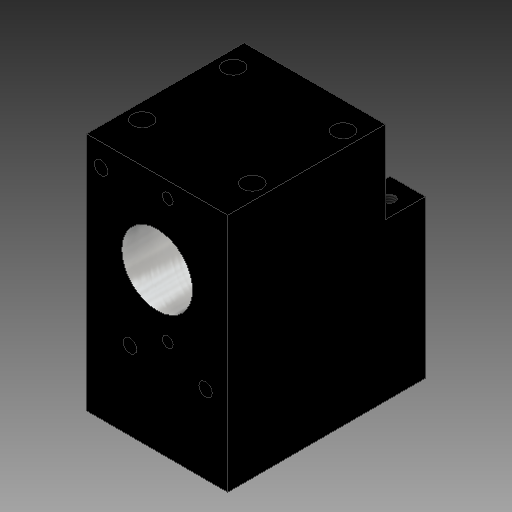
# Autodesk Inventor part: J007515
Saved by Autodesk Inventor 2018.2 (Build 222227000, 227)
## iProperties
Created: 2018-06-06
Part Number: J007515
Material: ALUMINUM, 6061-T651
Document SubType Name: Modeling
Designer: legant_local
Density: 2.7 g/cm^3
Appearance: Anodized - Black
Catalog Web Link: MPFI custom
Description: ResGalvoMount_wobble
Vendor: HHMI: JRC - JET
Project: P-303502
ALTERED ITEM PART NUMBER: N/A
ALTERED ITEM VENDOR: N/A
ALTERED ITEM DESCRIPTION: N/A
DESIGN DEPARTMENT: HHMI: JRC - ID&F
LAB/DEPT: BETZIG (LAB)
REQUESTING SCIENTIST: BETZIG, ERIC
SPECIAL FINISH: ANODIZE PER MIL-A-8625F, TYPE II, CLASS 2 (BLACK)
SURFACE ROUGHNESS: 32 Ra
Author: legant_local
Revision Number: 0
Autodesk Inventor part; units mm, degrees
ref_plane "YZ Plane" through (0, 0, 0) normal (1, 0, 0) x (0, 1, 0)
ref_plane "XZ Plane" through (0, 0, 0) normal (0, 1, 0) x (-1, 0, 0)
ref_plane "XY Plane" through (0, 0, 0) normal (0, 0, 1) x (1, 0, 0)
sketch "Sketch1" plane through (0, 0, 0) normal (0, 0, 1) x (1, 0, 0)
  line L0 (-15.875, 18.975) -> (15.875, 18.975)
  line L1 (15.875, 18.975) -> (15.875, -35)
  line L2 (15.875, -35) -> (-15.875, -35)
  line L3 (-15.875, -35) -> (-15.875, 18.975)
  point P0 (0, 0)
  dimension "d0" = 31.75
  dimension "d1" = 53.975
  dimension "d3" = 35
  dimension "d4" = 15.875
  constraints: 8 end point, 2 parallel, 1 horizontal, 1 perpendicular
  measures "d0" distance of L1.end L2.end
  measures "d1" distance of L0.end L1.end
  measures "d3" distance from line of L2 point (0, 0)
  measures "d4" distance from line of L3 point (0, 0)
extrude "Extrusion1" add sketch "Sketch1" along normal blind 44.45
sketch "Sketch2" plane through (0, 0, 44.45) normal (0, 0, 1) x (1, 0, 0)
  circle A0 centre (0, 0.3862) radius 7.9629
  line L0 (15.875, 18.975) -> (-15.875, 18.975) projected
  line L1 (-15.875, 18.975) -> (-15.875, -35) projected
  line L2 (-15.875, -35) -> (15.875, -35) projected
  line L3 (15.875, -35) -> (15.875, 18.975) projected
  line L4 (15.875, 18.975) -> (-15.875, 18.975) projected
  line L5 (0, 18.975) -> (0, -35) construction
  dimension "d7" = 15.9258
  dimension "d124" = 35.3862
  constraints: 2 end point, 2 midpoint, 1 centre point, 1 point on line
  measures "d7" diameter of A0
  measures "d124" distance from line of L2 A0.centre
extrude "Extrusion2" cut sketch "Sketch2" against normal through all contours A0
sketch "Sketch4" plane through (-15.875, 18.975, 0) normal (0, 1, 0) x (1, 0, 0)
  line L0 (0, 0) -> (31.75, 0) projected
  line L1 (31.75, 0) -> (0, 0)
  line L2 (0, 0) -> (0, -9)
  line L3 (0, -9) -> (31.75, -9)
  line L4 (31.75, -9) -> (31.75, 0)
  line L5 (0, 0) -> (0, -44.45) projected
  point P0 (15.875, 0)
  point P1 (0, -4.5)
  dimension "d15" = 9
  constraints: 8 end point, 2 parallel, 1 horizontal, 1 midpoint, 1 perpendicular, 1 point on line
  measures "d15" distance of L3.end L0.end
extrude "Extrusion4" cut sketch "Sketch4" against normal blind 18.5888
sketch "Sketch6" plane through (0, 0, 44.45) normal (0, 0, 1) x (1, 0, 0)
  line L0 (15.875, -15.95) -> (-11.125, -15.95) projected
  line L1 (-11.125, -15.95) -> (-11.125, 18.975) projected
  point P0 (0, 0)
  point P1 (-6.125, -17.45)
  point P2 (10.875, -17.45)
  point P3 (-12.625, 13.975)
  dimension "d33" = 1.5
  dimension "d34" = 1.5
  dimension "d35" = 5
  dimension "d36" = 5
  dimension "d44" = 5
  dimension "d45" = 1.5
  measures "d33" distance from line of L0 point (10.875, -17.45)
  measures "d34" distance from line of L0 point (-6.125, -17.45)
  measures "d35" horizontal distance of point (-6.125, -17.45) L0.end
  measures "d36" horizontal distance of L0.start point (10.875, -17.45)
  measures "d44" vertical distance of L1.end point (-12.625, 13.975)
  measures "d45" distance from line of L1 point (-12.625, 13.975)
hole "Press fit for D3mm_L10mm Dowel - pin to protrude 5mm" at (-6.125, -17.45, 44.45) at (10.875, -17.45, 44.45) at (-12.625, 13.975, 44.45) direction (0, 0, -1) diameter 3 depth 5 tip angle 118
sketch "Sketch9" plane through (-15.875, 18.975, 44.45) normal (0, 1, 0) x (1, 0, 0)
  line L0 (31.75, 35.45) -> (0, 35.45) projected
  line L1 (0, 35.45) -> (0, 0) projected
  line L2 (31.75, 0) -> (0, 0) projected
  line L3 (31.75, 35.45) -> (31.75, 0) projected
  line L4 (23.8379, 35.45) -> (23.8379, 44.45) projected
  line L5 (7.9121, 44.45) -> (23.8379, 44.45) projected
  line L6 (7.9121, 44.45) -> (7.9121, 35.45) projected
  line L7 (7.9121, 35.45) -> (23.8379, 35.45) projected
  line L8 (23.8379, 0) -> (7.9121, 0) projected
  point P0 (15.875, 44.45)
  point P1 (28.25, 9)
  point P2 (3.5, 9)
  point P3 (3.5, 29.45)
  point P4 (28.25, 29.45)
  dimension "d60" = 9
  dimension "d61" = 3.5
  dimension "d62" = 3.5
  dimension "d63" = 9
  dimension "d96" = 6
  dimension "d97" = 6
  dimension "d98" = 3.5
  dimension "d99" = 3.5
  measures "d60" distance from line of L2 point (28.25, 9)
  measures "d61" distance from line of L3 point (28.25, 9)
  measures "d62" distance from line of L1 point (3.5, 9)
  measures "d63" distance from line of L2 point (3.5, 9)
  measures "d96" distance from line of L0 point (3.5, 29.45)
  measures "d97" distance from line of L0 point (28.25, 29.45)
  measures "d98" distance from line of L3 point (28.25, 29.45)
  measures "d99" distance from line of L1 point (3.5, 29.45)
hole "Cbore hole for M2 screw_1" at (12.375, 18.975, 35.45) at (-12.375, 18.975, 35.45) at (-12.375, 18.975, 15) at (12.375, 18.975, 15) direction (0, -1, 0) diameter 2.4 end through all counterbore diameter 4.4 counterbore depth 39 clearance for "Socket Head Cap Screw" size "M2" standard "Ansi Metric M Profile"
sketch "Sketch11" plane through (15.875, 18.975, 9) normal (0, 0, -1) x (-1, 0, 0)
  circle A0 centre (13.5, -3.5) radius 0.7835 projected
  point P0 (15.875, -18.975)
hole "Cbore hole for M2 screw_2" at (2.375, 15.475, 9) direction (0, 0, 1) diameter 2.4 end through all counterbore diameter 4.4 counterbore depth 20 clearance for "Socket Head Cap Screw" size "M2" standard "Ansi Metric M Profile"
sketch "Sketch12" plane through (0, 0, 0) normal (0, 0, -1) x (-1, 0, 0)
  circle A0 centre (-2.375, -12.45) radius 0.7835 projected
  point P0 (0, 0)
hole "Cbore hole for M2 screw_3" at (2.375, -12.45, 0) direction (0, 0, 1) diameter 2.4 end through all counterbore diameter 4.4 counterbore depth 29 clearance for "Socket Head Cap Screw" size "M2" standard "Ansi Metric M Profile"
sketch "Sketch13" plane through (-15.875, -35, 0) normal (0, -1, 0) x (1, 0, 0)
  circle A0 centre (3.5, 15) radius 1.2 projected
  circle A1 centre (28.25, 35.45) radius 1.2 projected
  circle A2 centre (3.5, 35.45) radius 1.2 projected
  circle A3 centre (28.25, 15) radius 1.2 projected
  line L0 (31.75, 0) -> (0, 0) projected
  line L1 (31.75, 0) -> (31.75, 44.45) projected
  line L2 (0, 44.45) -> (31.75, 44.45) projected
  line L3 (0, 0) -> (0, 44.45) projected
  line L4 (0, 44.45) -> (31.75, 44.45) projected
  line L5 (20.45, 0) -> (16.05, 0) projected
  line L6 (15.875, 44.45) -> (15.875, 0) construction
  point P0 (15.875, 0)
  point P1 (15.875, 38.45)
  point P2 (15.875, 6)
  dimension "d100" = 6
  dimension "d101" = 6
  constraints: 2 end point, 2 midpoint, 2 point on line, 1 vertical
  measures "d100" distance from line of L2 point (15.875, 38.45)
  measures "d101" distance from line of L0 point (15.875, 6)
hole "Locating Holes for Mitsumi CJPDB3-4" at (0, -35, 38.45) at (0, -35, 6) direction (0, 1, 0) diameter 4 depth 8 tip angle 118 countersink diameter 5 countersink angle 90
sketch "Sketch15" plane through (-15.875, 0.3862, 0) normal (0, 1, 0) x (1, 0, 0)
  circle A0 centre (3.556, -4.445) radius 1.7 projected
  circle A1 centre (28.194, -4.445) radius 1.7 projected
  point P0 (15.875, 0)
hole "Threaded hole for M3 screw" at (12.319, 0.3862, 4.445) at (-12.319, 0.3862, 4.445) direction (0, -1, 0) diameter 2.459 depth 10 tip angle 118 thread size "M3x0.5" class "6H" standard "ANSI Metric M Profile"
equation "\"d4\" = 0.5 * d0"
body "Solid1"
